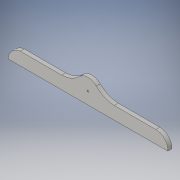
# Autodesk Inventor part: holder
Saved by Autodesk Inventor 2016 (Build 200138000, 138)
## iProperties
Created: 2017-12-14
Part Number: holder
Material: Generic
Document SubType Name: Modeling
Designer: student
Density: 1 g/cm^3
Appearance: Default
Author: student
Autodesk Inventor part; units mm, degrees
ref_plane "YZ Plane" through (0, 0, 0) normal (1, 0, 0) x (0, 1, 0)
ref_plane "XZ Plane" through (0, 0, 0) normal (0, 1, 0) x (-1, 0, 0)
ref_plane "XY Plane" through (0, 0, 0) normal (0, 0, 1) x (1, 0, 0)
sketch "Sketch1" plane through (0, 0, 0) normal (0, 0, 1) x (1, 0, 0)
  line L0 (0, 0) -> (254, 0)
  circle A0 centre (127, 20.32) radius 9.652 construction
  line L1 (127, 38.1) -> (127, 0) construction
  arc A1 (85.2807, 20.21) -> (113.8319, 32.6419) centre (83.7743, 62.6708) ccw
  arc A2 (127, 38.1) -> (113.8319, 32.6419) centre (127, 19.4864) ccw
  arc A3 (140.1681, 32.6419) -> (168.7193, 20.21) centre (170.2257, 62.6708) ccw
  arc A4 (140.1681, 32.6419) -> (127, 38.1) centre (127, 19.4864) ccw
  line L2 (85.2807, 20.21) -> (19.2407, 20.21)
  line L3 (168.7193, 20.21) -> (234.7593, 20.21)
  arc A5 (254, 0) -> (234.7593, 20.21) centre (234.7593, 0.9461) ccw
  arc A6 (19.2407, 20.21) -> (0, 0) centre (21.9577, -1.6406) ccw
  dimension "d2" = 19.304
  dimension "d74" = 254
  dimension "d75" = 20.32
  dimension "d76" = 38.1
  dimension "d78" = 42.4876
  dimension "d79" = 18.6136
  dimension "d89" = 66.04
  dimension "d90" = 66.04
  dimension "d91" = 22.0189
  dimension "d92" = 19.2639
  dimension "d93" = 21.8506
  constraints: 12 point on circle, 8 end point, 7 centre point, 4 symmetric about line, 3 horizontal, 3 tangent, 1 coincident, 1 horizontal alignment, 1 midpoint, 1 vertical, 1 vertical alignment, 2 other
  measures "d2" diameter of A0
  measures "d74" distance of L0.start L0.end
  measures "d75" distance from line of L0 A0.centre
  measures "d76" distance of L1.start L1.end
  measures "d78" radius of A1
  measures "d79" radius of A2
  measures "d89" distance of L2.start L2.end
  measures "d90" distance of L3.start L3.end
  measures "d91" radius of A6
  measures "d92" radius of A5
  measures "d93" distance from line of A6.centre L2
extrude "Extrusion2" add sketch "Sketch1" along normal blind 6.35
sketch "Sketch5" plane through (0, 0, 6.35) normal (0, 0, 1) x (1, 0, 0)
  circle A0 centre (127, 19.05) radius 9.652
  line L0 (0, 0) -> (254, 0) projected
  arc A1 (140.1681, 32.6419) -> (113.8319, 32.6419) centre (127, 19.4864) ccw projected
  point P0 (127, 1.27)
  point P1 (127, 38.1)
  dimension "d58" = 19.304
  dimension "d87" = 19.05
  constraints: 2 vertical alignment, 1 centre point, 1 point on circle
  measures "d58" diameter of A0
  measures "d87" distance from line of L0 A0.centre
hole "Hole3" at (127, 19.05, 6.35) direction (0, 0, -1) diameter 2.54 end through all
body "Solid2"
